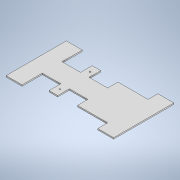
# Autodesk Inventor part: onderkant
Saved by Autodesk Inventor 2022 (Build 260153000, 153)
## iProperties
Created: 2021-12-16
Part Number: onderkant
Material: Generic
Document SubType Name: Modeling
Designer: keemi
Density: 1 g/cm^3
Appearance: Default
Author: keemi
Autodesk Inventor part; units mm, degrees
ref_plane "YZ Plane" through (0, 0, 0) normal (1, 0, 0) x (0, 1, 0)
ref_plane "XZ Plane" through (0, 0, 0) normal (0, 1, 0) x (-1, 0, 0)
ref_plane "XY Plane" through (0, 0, 0) normal (0, 0, 1) x (1, 0, 0)
sketch "Sketch1" plane through (0, 0, 0) normal (0, 1, 0) x (-1, 0, 0)
  line L0 (0, 0) -> (250, 0)
  line L1 (250, 0) -> (250, -140)
  line L2 (250, -140) -> (0, -140)
  line L3 (0, -140) -> (0, 0)
  dimension "d0" = 250
  dimension "d1" = 140
  constraints: 8 end point, 2 parallel, 1 horizontal, 1 perpendicular
  measures "d0" distance of L1.end L2.end
  measures "d1" distance of L0.end L1.end
extrude "Extrusion1" add sketch "Sketch1" along normal blind 3
sketch "Sketch2" plane through (0, 3, 0) normal (0, 1, 0) x (1, 0, 0)
  line L0 (-250, 140) -> (-250, 0) projected
  line L1 (-250, 0) -> (-160, 0)
  line L2 (-250, 0) -> (0, 0) projected
  line L3 (-160, 0) -> (-160, 20)
  line L4 (-160, 0) -> (-150, 0)
  line L5 (-150, 0) -> (-170, 0)
  line L6 (-170, 0) -> (-170, 20)
  line L7 (-170, 20) -> (-150, 20)
  line L8 (-150, 20) -> (-150, 0)
  line L9 (-170, 0) -> (-213, 0)
  line L10 (-213, 0) -> (-213, 47)
  line L11 (-213, 47) -> (-170, 47)
  line L12 (-170, 47) -> (-170, 0)
  line L13 (-150, 0) -> (-107, 0)
  line L14 (-107, 0) -> (-107, 47)
  line L15 (-107, 47) -> (-150, 47)
  line L16 (-150, 47) -> (-150, 0)
  line L17 (-170, 47) -> (-170, 140)
  line L18 (0, 140) -> (-250, 140) projected
  line L19 (-170, 140) -> (-213, 140)
  line L20 (-213, 140) -> (-213, 93)
  line L21 (-213, 93) -> (-170, 93)
  line L22 (-170, 93) -> (-170, 140)
  line L23 (-170, 140) -> (-150, 140)
  line L24 (-150, 140) -> (-150, 120)
  line L25 (-150, 120) -> (-170, 120)
  line L26 (-170, 120) -> (-170, 140)
  line L27 (-150, 140) -> (-107, 140)
  line L28 (-107, 140) -> (-107, 93)
  line L29 (-107, 93) -> (-150, 93)
  line L30 (-150, 93) -> (-150, 140)
  point P0 (-213, 0)
  point P1 (-107, 0)
  point P2 (-213, 140)
  point P3 (-170, 93)
  dimension "d4" = 90
  dimension "d5" = 20
  dimension "d6" = 10
  dimension "d7" = 20
  dimension "d8" = 20
  dimension "d9" = 43
  dimension "d10" = 47
  dimension "d11" = 43
  dimension "d12" = 47
  dimension "d31" = 43
  dimension "d32" = 47
  dimension "d33" = 20
  dimension "d34" = 20
  dimension "d35" = 43
  dimension "d36" = 47
  constraints: 56 end point, 12 parallel, 7 perpendicular, 6 horizontal, 3 point on line, 1 vertical
  measures "d4" distance of L0.end L1.end
  measures "d5" distance of L1.end L3.end
  measures "d6" distance of L1.end L4.end
  measures "d7" distance of L6.end L7.end
  measures "d8" distance of L5.end L6.end
  measures "d9" distance of L10.end L11.end
  measures "d10" distance of L9.end L10.end
  measures "d11" distance of L15.end L14.end
  measures "d12" distance of L14.end L13.end
  measures "d31" distance of L21.end L20.end
  measures "d32" distance of L20.end L19.end
  measures "d33" distance of L24.end L25.end
  measures "d34" distance of L23.end L24.end
  measures "d35" distance of L28.end L29.end
  measures "d36" distance of L27.end L28.end
extrude "Extrusion2" cut sketch "Sketch2" against normal blind 50 contours L18 L17 L21 L20 | L10 L11 L12 L6 L1 | L18 L24 L25 L17 | L6 L7 L3 L1 | L18 L28 L29 L30 L24 | L3 L7 L8 L2 | L8 L16 L15 L14 L2
sketch "Sketch3" plane through (0, 3, 0) normal (0, 1, 0) x (1, 0, 0)
  line L0 (-170, 20) -> (-170, 47) projected
  line L1 (-170, 20) -> (-160, 20)
  line L2 (-170, 20) -> (-150, 20) projected
  line L3 (-160, 20) -> (-160, 35)
  line L4 (-170, 120) -> (-150, 120) projected
  line L5 (-170, 120) -> (-160, 120)
  line L6 (-160, 120) -> (-160, 105)
  point P0 (0, 0)
  dimension "d21" = 15
  dimension "d29" = 10
  dimension "d30" = 15
  constraints: 8 end point, 2 midpoint, 1 perpendicular, 1 vertical
  measures "d21" distance of L1.end L3.end
  measures "d29" distance of L4.start L5.end
  measures "d30" distance of L5.end L6.end
hole "Hole1" at (-160, 3, -35) at (-160, 3, -105) direction (0, -1, 0) diameter 3 end through all
sketch "Sketch4" plane through (0, 3, 0) normal (0, 1, 0) x (1, 0, 0)
  line L0 (-107, 0) -> (0, 0) projected
  line L1 (-107, 0) -> (-37, 0)
  line L2 (-37, 0) -> (-37, 23)
  line L3 (-37, 23) -> (-107, 23)
  line L4 (-107, 23) -> (-107, 0)
  line L5 (0, 140) -> (-107, 140) projected
  line L6 (-107, 140) -> (-37, 140)
  line L7 (-37, 140) -> (-37, 117)
  line L8 (-37, 117) -> (-107, 117)
  line L9 (-107, 117) -> (-107, 140)
  dimension "d37" = 70
  dimension "d38" = 23
  dimension "d39" = 70
  dimension "d40" = 23
  constraints: 16 end point, 4 parallel, 2 horizontal, 2 perpendicular
  measures "d37" distance of L3.end L2.end
  measures "d38" distance of L2.end L1.end
  measures "d39" distance of L7.end L8.end
  measures "d40" distance of L6.end L7.end
extrude "Extrusion3" cut sketch "Sketch4" against normal blind 50
equation "\"d9\" = d11"
equation "\"d10\" = d12"
equation "\"d31\" = d35"
equation "\"d32\" = d36"
equation "\"d35\" = d11"
equation "\"d36\" = d12"
equation "\"d13\" = d16"
equation "\"d41\" = d16"
equation "\"d16\" = 50"
body "Solid1"
